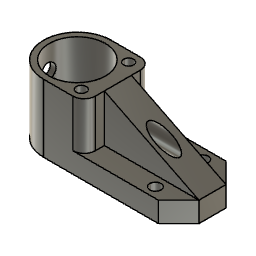
My First Projects (Autodesk Fusion 360 design; units mm, degrees)
Autodesk Fusion 360 part; units mm, degrees
sketch "Sketch1" plane through (0, 0, 0) normal (0, 1, 0) x (1, 0, 0)
sketch "Sketch2" plane through (0, 0, 0) normal (0, 0, 1) x (1, 0, 0)
  line L0 (30, 15) -> (-30, 15)
  line L1 (-30, 15) -> (-30, -15)
  line L2 (-30, -15) -> (30, -15)
  line L3 (30, -15) -> (30, 15)
  line L4 (30, 15) -> (-30, -15) construction
  line L5 (-30, 15) -> (30, -15) construction
  arc A0 (-30, 15) -> (-30, -15) centre (-30, 0) ccw
  circle A1 centre (-30, 0) radius 7.5
  line L6 (21, -15) -> (30, -6)
  line L7 (21, 15) -> (30, 6)
  dimension "d1" = 60
  dimension "d2" = 30
  dimension "d3" = 15
  dimension "d4" = 9
  dimension "d5" = 9
  dimension "d6" = 9
  dimension "d7" = 9
  constraint horizontal L0
  constraint perpendicular L0 L1
  constraint parallel L0 L2
  constraint parallel L1 L3
  constraint coincident L4 origin
  constraint coincident L5 origin
  constraint midpoint L1 A0.centre
  constraint concentric A0 A1
  constraint coincident L2 L6.start
  constraint coincident L3 L6.end
  constraint coincident L0 L7.start
  constraint coincident L3 L7.end
  measures "d1" distance of L1.end L2.end
  measures "d2" distance of L0.end L1.end
  measures "d3" diameter of A1
  measures "d4" distance of L2.end L6.start
  measures "d5" distance of L2.end L6.end
  measures "d6" distance of L0.start L7.start
  measures "d7" distance of L0.start L7.end
extrude "Extrude1" add sketch "Sketch2" along normal blind 9 contours L0 L1 L2 L3 A1 L6 L7 | L1 A0 A1
sketch "Sketch3" plane through (0, 0, 9) normal (0, 0, 1) x (-1, 0, 0)
  circle A0 centre (30, 0) radius 7.5
  arc A1 (30, -15) -> (30, 15) centre (30, 0) ccw
  line L0 (30, 15) -> (-21, 15)
  line L1 (-21, 15) -> (-30, 6)
  line L2 (-30, 6) -> (-30, -6)
  line L3 (-30, -6) -> (-21, -15)
  line L4 (-21, -15) -> (30, -15)
  line L5 (12, 15) -> (12, -15)
  dimension "d10" = 18
  constraint coincident L0 L5.start
  constraint coincident L4 L5.end
  constraint perpendicular L4 L5
  measures "d10" distance of A0.centre L5
extrude "Extrude2" add sketch "Sketch3" along normal blind 21 contours A1 L0 L4 L5
sketch "Sketch4" plane through (0, 0, 0) normal (0, 1, 0) x (1, 0, 0)
  line L0 (30, -9) -> (-12, -30)
  line L1 (-12, -30) -> (-12, -9)
  line L2 (-12, -9) -> (30, -9)
  constraint vertical L1
  constraint perpendicular L1 L2
extrude "Extrude3" add sketch "Sketch4" along normal mid plane 12
sketch "Sketch5" plane through (0, 0, 30) normal (0, 0, 1) x (-1, 0, 0)
  circle A0 centre (30, 0) radius 7.5
  line L0 (12, 15) -> (12, 6)
  line L1 (12, 6) -> (12, -6)
  line L2 (12, -6) -> (12, -15)
  line L3 (12, -15) -> (30, -15)
  arc A1 (30, -15) -> (30, 15) centre (30, 0) ccw
  line L4 (30, 15) -> (12, 15)
  circle A2 centre (17.7307, -10.5) radius 2.2228
  circle A3 centre (17.7307, -10.5) radius 2.5
  dimension "d15" = 5
  constraint concentric A2 A3
  measures "d15" diameter of A3
extrude "Extrude4" cut sketch "Sketch5" against normal blind 30 contours A2
mirror "Mirror1" about plane through (0, 0, 0) normal (0, 1, 0) of "Extrude4"
sketch "Sketch6" plane through (0, 0, 30) normal (0, 0, 1) x (-1, 0, 0)
  circle A0 centre (17.7307, 10.5) radius 2.2228
  circle A1 centre (17.7307, -10.5) radius 2.2228
  circle A2 centre (30, 0) radius 7.5
  line L0 (12, 15) -> (12, 6)
  line L1 (12, 6) -> (12, -6)
  line L2 (12, -6) -> (12, -15)
  line L3 (12, -15) -> (30, -15)
  arc A3 (30, -15) -> (30, 15) centre (30, 0) ccw
  line L4 (30, 15) -> (12, 15)
  circle A4 centre (30, 0) radius 12.5
  dimension "d20" = 25
  constraint concentric A2 A4
  measures "d20" diameter of A4
extrude "Extrude5" cut sketch "Sketch6" against normal blind 25 contours A4
sketch "Sketch7" plane through (0, 0, 5) normal (0, 0, 1) x (-1, 0, 0)
  circle A0 centre (30, 0) radius 7.5
  circle A1 centre (30, 0) radius 12.5
  circle A2 centre (30, 10) radius 1.25
  dimension "d23" = 2.5
  measures "d23" diameter of A2
extrude "Extrude6" cut sketch "Sketch7" against normal blind 5 contours A2
sketch "Sketch8" plane through (0, 0, 5) normal (0, 0, 1) x (-1, 0, 0)
  circle A0 centre (30, 10) radius 1.25
  circle A1 centre (30, 0) radius 7.5
  circle A2 centre (30, 0) radius 12.5
  circle A3 centre (30, -10) radius 1.25
  dimension "d26" = 2.5
  measures "d26" diameter of A3
extrude "Extrude7" cut sketch "Sketch8" against normal blind 5 contours A3
sketch "Sketch9" plane through (0, 0, 0) normal (0, 0, -1) x (1, 0, 0)
  circle A0 centre (-30, -10) radius 1.25
  circle A1 centre (-30, 10) radius 1.25
  circle A2 centre (-17.7307, 10.5) radius 2.2228
  circle A3 centre (-17.7307, -10.5) radius 2.2228
  circle A4 centre (-30, 0) radius 7.5
  arc A5 (-30, 15) -> (-30, -15) centre (-30, 0) ccw
  line L0 (-30, -15) -> (21, -15)
  line L1 (21, -15) -> (30, -6)
  line L2 (30, -6) -> (30, 6)
  line L3 (30, 6) -> (21, 15)
  line L4 (21, 15) -> (-30, 15)
  circle A6 centre (15.1822, -10.5) radius 2.5
  circle A7 centre (15, 10) radius 2.5
  dimension "d29" = 5
  dimension "d30" = 5
  measures "d29" diameter of A6
  measures "d30" diameter of A7
extrude "Extrude8" cut sketch "Sketch9" against normal blind 9 contours A6
mirror "Mirror2" about plane through (0, 0, 0) normal (0, 1, 0) of "Extrude8"
sketch "Sketch10" plane through (0, 0, 0) normal (0, 0, 1) x (1, 0, 0)
fillet "Fillet1" radius 5 1 edges at (-12, 15, 19.5)
fillet "Fillet2" radius 5 1 edges at (-12, -15, 19.5)
ref_plane "WorkPlane1" through (-57, -8, 19.5) normal (1, 0, 0) x (0, 1, 0)
sketch "Sketch11" plane through (-57, -8, 19.5) normal (1, 0, 0) x (0, 1, 0)
  circle A0 centre (7.2624, -0.0862) radius 3.5
  dimension "d40" = 7
  measures "d40" diameter of A0
extrude "Extrude9" cut sketch "Sketch11" along normal blind 75
